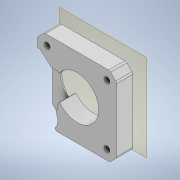
# Autodesk Inventor part: E-Motor Mount P1.0
Saved by Autodesk Inventor 2020 (Build 240168000, 168)
## iProperties
Created: 2019-11-15
Part Number: E-Motor Mount P1.0
Material: Generic
Document SubType Name: Modeling
Designer: pepd9
Density: 1 g/cm^3
Appearance: Default
Author: pepd9
Autodesk Inventor part; units mm, degrees
ref_plane "YZ Plane" through (0, 0, 0) normal (1, 0, 0) x (0, 1, 0)
ref_plane "XZ Plane" through (0, 0, 0) normal (0, 1, 0) x (-1, 0, 0)
ref_plane "XY Plane" through (0, 0, 0) normal (0, 0, 1) x (1, 0, 0)
sketch "Sketch1" plane through (0, 0, 0) normal (0, 0, 1) x (1, 0, 0)
  line L0 (20.0607, 17.4322) -> (17.4322, 20.0607) projected
  arc A0 (17.4322, 20.0607) -> (16.3716, 20.5) centre (16.3716, 19) ccw projected
  line L1 (16.3716, 20.5) -> (-16.3716, 20.5) projected
  arc A1 (-16.3716, 20.5) -> (-17.4322, 20.0607) centre (-16.3716, 19) ccw projected
  line L2 (-17.4322, 20.0607) -> (-20.0607, 17.4322) projected
  arc A2 (-20.0607, 17.4322) -> (-20.5, 16.3716) centre (-19, 16.3716) ccw projected
  line L3 (-20.5, 16.3716) -> (-20.5, -16.3716) projected
  arc A3 (-20.5, -16.3716) -> (-20.0607, -17.4322) centre (-19, -16.3716) ccw projected
  line L4 (-20.0607, -17.4322) -> (-17.4322, -20.0607) projected
  arc A4 (-17.4322, -20.0607) -> (-16.3716, -20.5) centre (-16.3716, -19) ccw projected
  line L5 (-16.3716, -20.5) -> (16.3716, -20.5) projected
  arc A5 (16.3716, -20.5) -> (17.4322, -20.0607) centre (16.3716, -19) ccw projected
  line L6 (17.4322, -20.0607) -> (20.0607, -17.4322) projected
  arc A6 (20.0607, -17.4322) -> (20.5, -16.3716) centre (19, -16.3716) ccw projected
  line L7 (20.5, -16.3716) -> (20.5, 16.3716) projected
  arc A7 (20.5, 16.3716) -> (20.0607, 17.4322) centre (19, 16.3716) ccw projected
  circle A8 centre (0, 0) radius 16.5 projected
  circle A9 centre (15.5, 15.5) radius 1.55 projected
  circle A10 centre (15.5, -15.5) radius 1.55 projected
  circle A11 centre (-15.5, -15.5) radius 1.55 projected
  circle A12 centre (-15.5, 15.5) radius 1.55 projected
  circle A13 centre (0, 0) radius 11.2
  point P0 (0, 0)
  point P1 (-20.0607, -17.4322)
  point P2 (20.0607, -17.4322)
  dimension "d0" = 22.4
  constraints: 1 centre point, 1 coincident
  measures "d0" diameter of A13
ref_plane "Work Plane1" through (-2, -20.5, 10.7) normal (0, 0, -1) x (0, 1, 0)
extrude "Extrusion1" add sketch "Sketch1" along normal blind 13.4 contours A7 L7 A6 L6 A5 L5 A4 L4 A3 L3 A2 L2 A1 L1 A0 L0 | A8
sketch "Sketch2" plane through (0, 0, 0) normal (0, 0, -1) x (-1, 0, 0)
  arc A0 (20.5, 16.3716) -> (20.0607, 17.4322) centre (19, 16.3716) ccw projected
  line L0 (17.4322, 20.0607) -> (20.0607, 17.4322) projected
  arc A1 (17.4322, 20.0607) -> (16.3716, 20.5) centre (16.3716, 19) ccw projected
  line L1 (-16.3716, 20.5) -> (16.3716, 20.5) projected
  arc A2 (-16.3716, 20.5) -> (-17.4322, 20.0607) centre (-16.3716, 19) ccw projected
  line L2 (-20.0607, 17.4322) -> (-17.4322, 20.0607) projected
  arc A3 (-20.0607, 17.4322) -> (-20.5, 16.3716) centre (-19, 16.3716) ccw projected
  line L3 (-20.5, -16.3716) -> (-20.5, 16.3716) projected
  arc A4 (-20.5, -16.3716) -> (-20.0607, -17.4322) centre (-19, -16.3716) ccw projected
  line L4 (-17.4322, -20.0607) -> (-20.0607, -17.4322) projected
  arc A5 (-17.4322, -20.0607) -> (-16.3716, -20.5) centre (-16.3716, -19) ccw projected
  line L5 (16.3716, -20.5) -> (-16.3716, -20.5) projected
  arc A6 (16.3716, -20.5) -> (17.4322, -20.0607) centre (16.3716, -19) ccw projected
  line L6 (20.0607, -17.4322) -> (17.4322, -20.0607) projected
  arc A7 (20.0607, -17.4322) -> (20.5, -16.3716) centre (19, -16.3716) ccw projected
  line L7 (20.5, 16.3716) -> (20.5, -16.3716) projected
  circle A8 centre (0, 0) radius 11.2 projected
  circle A9 centre (-15.5, 15.5) radius 1.55 projected
  circle A10 centre (15.5, -15.5) radius 1.55 projected
  circle A11 centre (-15.5, -15.5) radius 1.55 projected
  circle A12 centre (15.5, 15.5) radius 1.55 projected
  line L8 (8, -6) -> (9.4172, -7.0036) projected
  arc A13 (9.8231, -7.6405) -> (9.4172, -7.0036) centre (8.8393, -7.8197) ccw projected
  line L9 (10.3441, -10.5) -> (9.8231, -7.6405) projected
  line L10 (10.3441, -10.5) -> (15.5, -10.5) projected
  arc A14 (20.5, -15.5) -> (15.5, -10.5) centre (15.5, -15.5) ccw projected
  line L11 (20.5, 12.2) -> (20.5, -15.5) projected
  line L12 (19.3603, 12.2) -> (20.5, 12.2) projected
  line L13 (19.3603, 12.2) -> (13.3312, 6.9) projected
  line L14 (13.3312, 6.9) -> (10, 6.9) projected
  line L15 (10, 6.9) -> (9.0137, 5.9137) projected
  arc A15 (8, -6) -> (9.0137, 5.9137) centre (8, 0) ccw construction
  line L16 (10.3441, -10.5) -> (15.5, -10.5) projected
  line L17 (10.6868, -12.3805) -> (10.3441, -10.5) projected
  arc A16 (10.5948, -13.0121) -> (10.6868, -12.3805) centre (9.703, -12.5598) ccw projected
  arc A17 (10.5948, -13.0121) -> (11.1648, -18.8846) centre (15.5, -15.5) ccw projected
  arc A18 (10.3765, -20.5) -> (11.1648, -18.8846) centre (10.3765, -19.5) ccw projected
  line L18 (17, -20.5) -> (10.3765, -20.5) projected
  line L19 (17, -20.5) -> (20.5, -17) projected
  line L20 (20.5, -17) -> (20.5, -15.5) projected
  arc A19 (20.5, -15.5) -> (15.5, -10.5) centre (15.5, -15.5) ccw projected
  circle A20 centre (15.5, -15.5) radius 1.65 projected
  point P0 (0, 0)
  point P1 (9.3164, 6.2164)
  point P2 (8.9796, -6.6937)
extrude "Extrusion2" cut sketch "Sketch2" against normal through all contours L7 A14 L10 L9 A13 L8 A8 L15 L14 L13 L12 | L7 A7 L6 A6 L5 A18 A17 A16 L17 L10 A14 | A20
ref_plane "Work Plane2" through (0, 0, 0) normal (0, 0, 1) x (1, 0, 0)
sketch "Sketch3" plane through (0, 0, 0) normal (0, 0, 1) x (1, 0, 0)
  line L0 (20.0607, 17.4322) -> (17.4322, 20.0607) projected
  arc A0 (17.4322, 20.0607) -> (16.3716, 20.5) centre (16.3716, 19) ccw projected
  line L1 (16.3716, 20.5) -> (-16.3716, 20.5) projected
  arc A1 (-16.3716, 20.5) -> (-17.4322, 20.0607) centre (-16.3716, 19) ccw projected
  line L2 (-17.4322, 20.0607) -> (-20.0607, 17.4322) projected
  arc A2 (-20.0607, 17.4322) -> (-20.5, 16.3716) centre (-19, 16.3716) ccw projected
  line L3 (-20.5, 16.3716) -> (-20.5, -16.3716) projected
  arc A3 (-20.5, -16.3716) -> (-20.0607, -17.4322) centre (-19, -16.3716) ccw projected
  line L4 (-20.0607, -17.4322) -> (-17.4322, -20.0607) projected
  arc A4 (-17.4322, -20.0607) -> (-16.3716, -20.5) centre (-16.3716, -19) ccw projected
  line L5 (-16.3716, -20.5) -> (16.3716, -20.5) projected
  arc A5 (16.3716, -20.5) -> (17.4322, -20.0607) centre (16.3716, -19) ccw projected
  line L6 (17.4322, -20.0607) -> (20.0607, -17.4322) projected
  arc A6 (20.0607, -17.4322) -> (20.5, -16.3716) centre (19, -16.3716) ccw projected
  line L7 (20.5, -16.3716) -> (20.5, 16.3716) projected
  arc A7 (20.5, 16.3716) -> (20.0607, 17.4322) centre (19, 16.3716) ccw projected
  circle A8 centre (0, 0) radius 16.5 projected
  circle A9 centre (15.5, 15.5) radius 1.55 projected
  circle A10 centre (15.5, -15.5) radius 1.55 projected
  circle A11 centre (-15.5, -15.5) radius 1.55 projected
  circle A12 centre (-15.5, 15.5) radius 1.55 projected
  arc A13 (-11.1648, -18.8846) -> (-10.3765, -20.5) centre (-10.3765, -19.5) ccw projected
  line L8 (-10.3765, -20.5) -> (16.3716, -20.5) projected
  arc A14 (16.3716, -20.5) -> (17.4322, -20.0607) centre (16.3716, -19) ccw projected
  line L9 (17.4322, -20.0607) -> (20.0607, -17.4322) projected
  arc A15 (20.0607, -17.4322) -> (20.5, -16.3716) centre (19, -16.3716) ccw projected
  line L10 (20.5, -16.3716) -> (20.5, 16.3716) projected
  arc A16 (20.5, 16.3716) -> (20.0607, 17.4322) centre (19, 16.3716) ccw projected
  line L11 (20.0607, 17.4322) -> (17.4322, 20.0607) projected
  arc A17 (17.4322, 20.0607) -> (16.3716, 20.5) centre (16.3716, 19) ccw projected
  line L12 (16.3716, 20.5) -> (-16.3716, 20.5) projected
  arc A18 (-16.3716, 20.5) -> (-17.4322, 20.0607) centre (-16.3716, 19) ccw projected
  line L13 (-17.4322, 20.0607) -> (-20.0607, 17.4322) projected
  arc A19 (-20.0607, 17.4322) -> (-20.5, 16.3716) centre (-19, 16.3716) ccw projected
  line L14 (-20.5, 16.3716) -> (-20.5, 12.2) projected
  line L15 (-20.5, 12.2) -> (-19.3603, 12.2) projected
  line L16 (-19.3603, 12.2) -> (-13.3312, 6.9) projected
  line L17 (-13.3312, 6.9) -> (-10, 6.9) projected
  line L18 (-10, 6.9) -> (-9.3164, 6.2164) projected
  arc A20 (-8.9796, -6.6937) -> (-9.3164, 6.2164) centre (0, 0) ccw projected
  line L19 (-8.9796, -6.6937) -> (-9.4172, -7.0036) projected
  arc A21 (-9.4172, -7.0036) -> (-9.8231, -7.6405) centre (-8.8393, -7.8197) ccw projected
  line L20 (-9.8231, -7.6405) -> (-10.6868, -12.3805) projected
  arc A22 (-10.6868, -12.3805) -> (-10.5948, -13.0121) centre (-9.703, -12.5598) ccw projected
  arc A23 (-11.1648, -18.8846) -> (-10.5948, -13.0121) centre (-15.5, -15.5) ccw projected
  circle A24 centre (15.5, 15.5) radius 1.55 projected
  circle A25 centre (15.5, -15.5) radius 1.55 projected
  circle A26 centre (-15.5, 15.5) radius 1.55 projected
  point P0 (0, 0)
  point P1 (-10.703, -12.5577)
  point P2 (-14.4803, 7.9102)
  point P3 (-20.5, 12.2)
  point P4 (-17.4322, -20.0607)
  point P5 (-10.3765, -20.5)
extrude "Extrusion3" add sketch "Sketch3" along normal blind 5.7 contours L5 A4 L4 A3 L3 L15 L16 A8 A22 A23 A13
sketch "Sketch4" plane through (0, 0, 0) normal (0, 0, -1) x (-1, 0, 0)
  arc A0 (10.703, -12.5577) -> (10.6868, -12.3805) centre (9.703, -12.5598) ccw projected
  line L0 (10.6868, -12.3805) -> (9.8231, -7.6405) projected
  arc A1 (9.8231, -7.6405) -> (9.4172, -7.0036) centre (8.8393, -7.8197) ccw projected
  line L1 (9.4172, -7.0036) -> (8.9796, -6.6937) projected
  arc A2 (9.3164, 6.2164) -> (8.9796, -6.6937) centre (0, 0) ccw projected
  line L2 (9.3164, 6.2164) -> (10, 6.9) projected
  line L3 (10, 6.9) -> (13.3312, 6.9) projected
  line L4 (13.3312, 6.9) -> (14.4803, 7.9102) projected
  arc A3 (10.703, -12.5577) -> (14.4803, 7.9102) centre (0, 0) ccw projected
  circle A4 centre (15.5, -15.5) radius 1.55 projected
  circle A5 centre (15.5, 15.5) radius 1.55 projected
  circle A6 centre (-15.5, -15.5) radius 1.55 projected
  circle A7 centre (-15.5, 15.5) radius 1.55 projected
  line L5 (16.3716, -20.5) -> (-16.3716, -20.5) projected
  arc A8 (16.3716, -20.5) -> (17.4322, -20.0607) centre (16.3716, -19) ccw projected
  line L6 (20.0607, -17.4322) -> (17.4322, -20.0607) projected
  arc A9 (20.0607, -17.4322) -> (20.5, -16.3716) centre (19, -16.3716) ccw projected
  line L7 (20.5, 16.3716) -> (20.5, -16.3716) projected
  arc A10 (20.5, 16.3716) -> (20.0607, 17.4322) centre (19, 16.3716) ccw projected
  line L8 (17.4322, 20.0607) -> (20.0607, 17.4322) projected
  arc A11 (17.4322, 20.0607) -> (16.3716, 20.5) centre (16.3716, 19) ccw projected
  line L9 (-16.3716, 20.5) -> (16.3716, 20.5) projected
  arc A12 (-16.3716, 20.5) -> (-17.4322, 20.0607) centre (-16.3716, 19) ccw projected
  line L10 (-20.0607, 17.4322) -> (-17.4322, 20.0607) projected
  arc A13 (-20.0607, 17.4322) -> (-20.5, 16.3716) centre (-19, 16.3716) ccw projected
  line L11 (-20.5, -16.3716) -> (-20.5, 16.3716) projected
  arc A14 (-20.5, -16.3716) -> (-20.0607, -17.4322) centre (-19, -16.3716) ccw projected
  line L12 (-17.4322, -20.0607) -> (-20.0607, -17.4322) projected
  arc A15 (-17.4322, -20.0607) -> (-16.3716, -20.5) centre (-16.3716, -19) ccw projected
  point P0 (0, 0)
extrude "Extrusion4" cut sketch "Sketch4" against normal blind 5
body "Solid1"
